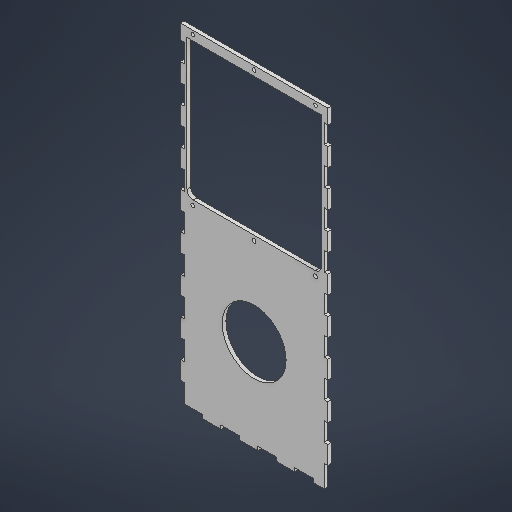
# Autodesk Inventor part: frente
Saved by Autodesk Inventor 2026 (Build 300175050, 175E)
## iProperties
Created: 2025-08-08
Part Number: frente
Material: Genérico
Document SubType Name: Modeling
Designer: EspacoMaker
Density: 1 g/cm^3
Appearance: Padrão
Author: EspacoMaker
Autodesk Inventor part; units mm, degrees
ref_plane "YZ Plane" through (0, 0, 0) normal (1, 0, 0) x (0, 1, 0)
ref_plane "XZ Plane" through (0, 0, 0) normal (0, 1, 0) x (-1, 0, 0)
ref_plane "XY Plane" through (0, 0, 0) normal (0, 0, 1) x (1, 0, 0)
sketch "Esboço1" plane through (0, 0, 0) normal (0, 0, 1) x (1, 0, 0)
  line L0 (60, -135) -> (-60, -135)
  line L1 (-60, -135) -> (-60, 135)
  line L2 (-60, 135) -> (60, 135)
  line L3 (60, 135) -> (60, -135)
  line L4 (60, -135) -> (-60, 135) construction
  line L5 (-60, -135) -> (60, 135) construction
  point P0 (0, 0)
  dimension "d0" = 120
  dimension "d1" = 270
  constraints: 12 end point, 2 midpoint, 2 parallel, 1 horizontal, 1 perpendicular
  measures "d0" distance of L1.end L2.end
  measures "d1" distance of L0.end L1.end
extrude "Extrusão1" add sketch "Esboço1" along normal blind 3
sketch "Esboço3" plane through (60, -135, 0) normal (1, 0, 0) x (0, 0, -1)
  line L0 (0, 0) -> (-3, 0) projected
  line L1 (0, 0) -> (-3, 0)
  line L2 (-3, 0) -> (-3, 18.1)
  line L3 (-3, 18.1) -> (0, 18.1)
  line L4 (0, 18.1) -> (0, 0)
  line L5 (-3, 2.9) -> (0, 2.9)
  line L6 (-3, 48.1) -> (0, 48.1)
  line L7 (-3, 32.9) -> (0, 32.9)
  line L8 (-3, 78.1) -> (0, 78.1)
  line L9 (-3, 62.9) -> (0, 62.9)
  line L10 (-3, 108.1) -> (0, 108.1)
  line L11 (-3, 92.9) -> (0, 92.9)
  line L12 (-3, 138.1) -> (0, 138.1)
  line L13 (-3, 122.9) -> (0, 122.9)
  line L14 (-3, 168.1) -> (0, 168.1)
  line L15 (-3, 152.9) -> (0, 152.9)
  line L16 (-3, 198.1) -> (0, 198.1)
  line L17 (-3, 182.9) -> (0, 182.9)
  line L18 (-3, 228.1) -> (0, 228.1)
  line L19 (-3, 212.9) -> (0, 212.9)
  line L20 (-3, 258.1) -> (0, 258.1)
  line L21 (-3, 242.9) -> (0, 242.9)
  line L22 (-3, 288.1) -> (0, 288.1)
  line L23 (-3, 272.9) -> (0, 272.9)
  line L24 (-3, 0) -> (-3, 270) projected
  line L25 (0, 0) -> (0, 270) projected
  point P0 (0, 135)
  dimension "d13" = 18.1
  dimension "d14" = 3
  dimension "d38" = 2.9
  dimension "d41" = 30
  constraints: 46 end point, 2 parallel, 2 perpendicular, 2 point on line, 1 horizontal, 1 vertical, 56 other
  measures "d13" distance of L1.end L2.end
  measures "d14" distance of L2.end L3.end
  measures "d38" distance between parallel lines of L0 L5
  measures "d41" distance of L2.end L6.start
extrude "Extrusão2" cut sketch "Esboço3" against normal blind 3 contours L0 L2 L5 L4 | L5 L2 L3 L4 | L7 L24 L6 L25 | L9 L24 L8 L25 | L11 L24 L10 L25 | L13 L24 L12 L25 | L15 L24 L14 L25 | L17 L24 L16 L25 | L19 L24 L18 L25 | L21 L24 L20 L25
sketch "Esboço5" plane through (57, -135, 0) normal (0, -1, 0) x (1, 0, 0)
  line L0 (-117, 0) -> (0, 0) projected
  line L1 (-114, 3) -> (-98.8, 3)
  line L2 (-98.8, 3) -> (-98.8, 0)
  line L3 (-98.8, 0) -> (-114, 0)
  line L4 (-114, 0) -> (-114, 3)
  line L5 (-84, 3) -> (-68.8, 3)
  line L6 (-68.8, 3) -> (-68.8, 0)
  line L7 (-68.8, 0) -> (-84, 0)
  line L8 (-84, 0) -> (-84, 3)
  line L9 (-54, 3) -> (-38.8, 3)
  line L10 (-38.8, 3) -> (-38.8, 0)
  line L11 (-38.8, 0) -> (-54, 0)
  line L12 (-54, 0) -> (-54, 3)
  line L13 (-24, 3) -> (-8.8, 3)
  line L14 (-8.8, 3) -> (-8.8, 0)
  line L15 (-8.8, 0) -> (-24, 0)
  line L16 (-24, 0) -> (-24, 3)
  line L17 (-117, 0) -> (-117, 3) projected
  point P0 (-57, 0)
  point P1 (-24, 0)
  point P2 (-54, 0)
  point P3 (-84, 0)
  point P4 (-117, 1.5)
  point P5 (-114, 1.5)
  dimension "d26" = 15.2
  dimension "d29" = 30
  dimension "d56" = 3
  constraints: 32 end point, 2 horizontal, 2 midpoint, 2 parallel, 1 collinear, 1 horizontal alignment, 1 perpendicular, 1 point on line, 23 other
  measures "d26" distance of L2.end L3.end
  measures "d29" distance of L2.end L6.end
  measures "d56" distance of point (-117, 1.5) point (-114, 1.5)
extrude "Extrusão4" cut sketch "Esboço5" against normal blind 3
sketch "Esboço7" plane through (-60, -135, 0) normal (-1, 0, 0) x (0, 0, 1)
  line L0 (3, 18.1) -> (0, 18.1) projected
  line L1 (3, 0) -> (3, 18.1) projected
  line L2 (0, 18.1) -> (0, 0) projected
  line L3 (0, 32.9) -> (3, 32.9) projected
  line L4 (3, 270) -> (3, 0) projected
  line L5 (0, 270) -> (0, 0) projected
  line L6 (0, 32.9) -> (3, 32.9)
  line L7 (0, 18.1) -> (3, 18.1)
  line L8 (0, 48.1) -> (3, 48.1)
  line L9 (0, 62.9) -> (3, 62.9)
  line L10 (0, 78.1) -> (3, 78.1)
  line L11 (0, 92.9) -> (3, 92.9)
  line L12 (0, 108.1) -> (3, 108.1)
  line L13 (0, 122.9) -> (3, 122.9)
  line L14 (0, 138.1) -> (3, 138.1)
  line L15 (0, 152.9) -> (3, 152.9)
  line L16 (0, 168.1) -> (3, 168.1)
  line L17 (0, 182.9) -> (3, 182.9)
  line L18 (0, 198.1) -> (3, 198.1)
  line L19 (0, 212.9) -> (3, 212.9)
  line L20 (0, 228.1) -> (3, 228.1)
  line L21 (0, 242.9) -> (3, 242.9)
  line L22 (0, 258.1) -> (3, 258.1)
  line L23 (0, 272.9) -> (3, 272.9)
  line L24 (0, 288.1) -> (3, 288.1)
  line L25 (0, 302.9) -> (3, 302.9)
  line L26 (3, 0) -> (0, 0) projected
  line L27 (0, 0) -> (0, 270) projected
  line L28 (0, 270) -> (3, 270) projected
  line L29 (3, 270) -> (3, 0) projected
  point P0 (0, 135)
  point P1 (3, 258.1)
  point P2 (0, 258.1)
  point P3 (0, 242.9)
  point P4 (3, 242.9)
  point P5 (3, 228.1)
  point P6 (0, 228.1)
  point P7 (0, 212.9)
  point P8 (3, 212.9)
  point P9 (3, 198.1)
  point P10 (0, 198.1)
  point P11 (0, 182.9)
  point P12 (3, 182.9)
  point P13 (3, 168.1)
  point P14 (0, 168.1)
  point P15 (0, 152.9)
  point P16 (3, 152.9)
  point P17 (3, 138.1)
  point P18 (0, 138.1)
  point P19 (0, 122.9)
  point P20 (3, 122.9)
  point P21 (3, 108.1)
  point P22 (0, 108.1)
  point P23 (0, 92.9)
  point P24 (3, 92.9)
  point P25 (3, 78.1)
  point P26 (0, 78.1)
  point P27 (0, 62.9)
  point P28 (3, 62.9)
  point P29 (3, 48.1)
  point P30 (0, 48.1)
  dimension "d49" = 30
  constraints: 40 end point, 2 horizontal, 1 vertical, 57 other
  measures "d49" distance of L0.end L8.start
extrude "Extrusão5" cut sketch "Esboço7" against normal blind 3 contours L1 L26 L2 L0 | L3 L5 L8 L4 | L9 L5 L10 L4 | L11 L5 L12 L4 | L13 L5 L14 L4 | L15 L5 L16 L4 | L17 L5 L18 L4 | L19 L5 L20 L4 | L21 L5 L22 L4
sketch "Esboço8" plane through (0, 0, 0) normal (0, 0, -1) x (-1, 0, 0)
  line L0 (-57, -86.9) -> (-60, -86.9) construction
  line L1 (-60, -86.9) -> (-60, -72.1) construction
  line L2 (-60, -72.1) -> (-57, -72.1) construction
  line L3 (-57, -72.1) -> (-57, -56.9) construction
  line L4 (-57, -56.9) -> (-60, -56.9) construction
  line L5 (-60, -56.9) -> (-60, -42.1) construction
  line L6 (-60, -42.1) -> (-57, -42.1) construction
  line L7 (-57, -42.1) -> (-57, -26.9) construction
  line L8 (-57, -26.9) -> (-60, -26.9) construction
  line L9 (-60, -26.9) -> (-60, -12.1) construction
  line L10 (-60, -12.1) -> (-57, -12.1) construction
  line L11 (-57, -12.1) -> (-57, 3.1) construction
  line L12 (-57, 3.1) -> (-60, 3.1) construction
  line L13 (-60, 3.1) -> (-60, 17.9) construction
  line L14 (-60, 17.9) -> (-57, 17.9) construction
  line L15 (-57, 17.9) -> (-57, 33.1) construction
  line L16 (-57, 33.1) -> (-60, 33.1) construction
  line L17 (-60, 33.1) -> (-60, 47.9) construction
  line L18 (-60, 47.9) -> (-57, 47.9) construction
  line L19 (-57, 47.9) -> (-57, 63.1) construction
  line L20 (-57, 63.1) -> (-60, 63.1) construction
  line L21 (-60, 63.1) -> (-60, 77.9) construction
  line L22 (-60, 77.9) -> (-57, 77.9) construction
  line L23 (-57, 77.9) -> (-57, 93.1) construction
  line L24 (-57, 93.1) -> (-60, 93.1) construction
  line L25 (-60, 93.1) -> (-60, 107.9) construction
  line L26 (-60, 107.9) -> (-57, 107.9) construction
  line L27 (-57, 107.9) -> (-57, 123.1) construction
  line L28 (-57, 123.1) -> (-60, 123.1) construction
  line L29 (-60, 123.1) -> (-60, 135) construction
  line L30 (-60, 135) -> (60, 135) construction
  line L31 (60, 135) -> (60, 123.1) construction
  line L32 (60, 123.1) -> (57, 123.1) construction
  line L33 (57, 123.1) -> (57, 107.9) construction
  line L34 (57, 107.9) -> (60, 107.9) construction
  line L35 (60, 107.9) -> (60, 93.1) construction
  line L36 (60, 93.1) -> (57, 93.1) construction
  line L37 (57, 93.1) -> (57, 77.9) construction
  line L38 (57, 77.9) -> (60, 77.9) construction
  line L39 (60, 77.9) -> (60, 63.1) construction
  line L40 (60, 63.1) -> (57, 63.1) construction
  line L41 (57, 63.1) -> (57, 47.9) construction
  line L42 (57, 47.9) -> (60, 47.9) construction
  line L43 (60, 47.9) -> (60, 33.1) construction
  line L44 (60, 33.1) -> (57, 33.1) construction
  line L45 (57, 33.1) -> (57, 17.9) construction
  line L46 (57, 17.9) -> (60, 17.9) construction
  line L47 (60, 17.9) -> (60, 3.1) construction
  line L48 (60, 3.1) -> (57, 3.1) construction
  line L49 (57, 3.1) -> (57, -12.1) construction
  line L50 (57, -12.1) -> (60, -12.1) construction
  line L51 (60, -12.1) -> (60, -26.9) construction
  line L52 (60, -26.9) -> (57, -26.9) construction
  line L53 (57, -26.9) -> (57, -42.1) construction
  line L54 (57, -42.1) -> (60, -42.1) construction
  line L55 (60, -42.1) -> (60, -56.9) construction
  line L56 (60, -56.9) -> (57, -56.9) construction
  line L57 (57, -56.9) -> (57, -72.1) construction
  line L58 (57, -72.1) -> (60, -72.1) construction
  line L59 (60, -72.1) -> (60, -86.9) construction
  line L60 (60, -86.9) -> (57, -86.9) construction
  line L61 (57, -86.9) -> (57, -102.1) construction
  line L62 (57, -102.1) -> (60, -102.1) construction
  line L63 (60, -102.1) -> (60, -116.9) construction
  line L64 (60, -116.9) -> (57, -116.9) construction
  line L65 (57, -116.9) -> (57, -132) construction
  line L66 (57, -132) -> (41.8, -132) construction
  line L67 (41.8, -132) -> (41.8, -135) construction
  line L68 (41.8, -135) -> (27, -135) construction
  line L69 (27, -135) -> (27, -132) construction
  line L70 (27, -132) -> (11.8, -132) construction
  line L71 (11.8, -132) -> (11.8, -135) construction
  line L72 (11.8, -135) -> (-3, -135) construction
  line L73 (-3, -135) -> (-3, -132) construction
  line L74 (-3, -132) -> (-18.2, -132) construction
  line L75 (-18.2, -132) -> (-18.2, -135) construction
  line L76 (-18.2, -135) -> (-33, -135) construction
  line L77 (-33, -135) -> (-33, -132) construction
  line L78 (-33, -132) -> (-48.2, -132) construction
  line L79 (-48.2, -132) -> (-48.2, -135) construction
  line L80 (-48.2, -135) -> (-57, -135) construction
  line L81 (-57, -135) -> (-57, -116.9) construction
  line L82 (-57, -116.9) -> (-60, -116.9) construction
  line L83 (-60, -116.9) -> (-60, -102.1) construction
  line L84 (-60, -102.1) -> (-57, -102.1) construction
  line L85 (-57, -102.1) -> (-57, -86.9) construction
  ellipse E0 centre (-55.4, 11.3042) end of major axis (-55.4, 8.4758) minor radius 2 (-57.4, 11.3042) -> (-57.1743, 9.9988) ccw
  line L86 (-57.1743, 9.9988) -> (59.4, 9.9988)
  line L87 (59.4, 127.5) -> (59.4, 9.9988)
  line L88 (-57.4, 127.5) -> (59.4, 127.5)
  line L89 (-57.4, 127.5) -> (-57.4, 11.3042)
  ellipse E1 centre (-56.5, 121.6939) end of major axis (-56.5, 127.5415) minor radius 2 (-54.5, 121.6939) -> (-55.7002, 127.0537) ccw
  line L90 (-55.7002, 127.0537) -> (55.7002, 127.0537)
  ellipse E2 centre (56.5, 121.6939) end of major axis (56.5, 127.5415) minor radius 2 (55.7002, 127.0537) -> (54.5, 121.6939) ccw
  line L91 (54.5, 121.6939) -> (54.5, 105.9054)
  line L92 (54.5, 105.9054) -> (49.5, 105.9054) construction
  line L93 (49.5, 105.9054) -> (49.5, 116.4119) construction
  line L94 (49.5, 116.4119) -> (-49.5, 116.4119) construction
  line L95 (-49.5, 116.4119) -> (-49.5, 105.9054) construction
  line L96 (-49.5, 105.9054) -> (-54.5, 105.9054) construction
  line L97 (-54.5, 105.9054) -> (-54.5, 121.6939)
  circle A0 centre (-50, 132) radius 1.5
  circle A1 centre (0, 132) radius 1.5
  circle A2 centre (50, 132) radius 1.5
  line L98 (60, 7.3988) -> (-60, 7.3988)
  line L99 (-60, 7.3988) -> (-60, 136)
  line L100 (-60, 136) -> (60, 136)
  line L101 (60, 136) -> (60, 7.3988)
  line L102 (-60, 7.3988) -> (60, 7.3988)
  line L103 (60, 7.3988) -> (60, 15.3988)
  line L104 (60, 15.3988) -> (-60, 15.3988)
  line L105 (-60, 15.3988) -> (-60, 7.3988)
  line L106 (-60, 11.3988) -> (60, 11.3988) construction
  circle A3 centre (0, 11.3988) radius 1.6
  circle A4 centre (-50, 11.3988) radius 1.6
  circle A5 centre (50, 11.3988) radius 1.6
  line L107 (54.5, 66.3189) -> (54.5, 124.5798)
  line L108 (-54.5, 124.5798) -> (-54.5, 66.3189)
  line L109 (-60, 136) -> (60, 136)
  line L110 (-60, 135) -> (60, 135) projected
  line L111 (-54.7, 15.3988) -> (-54.7, 127.5)
  line L112 (54.7, 127.5) -> (54.7, 15.3988)
  point P0 (-60, 49.3988)
  point P1 (54.7, 127.0537)
  point P2 (-54.7, 127.0537)
  point P3 (54.7, 124.2429)
  point P4 (-54.7, 124.2429)
  point P5 (-55.6594, 127)
  point P6 (55.6594, 127)
  point P7 (-49.2254, 9.9988)
  point P8 (-50.7746, 9.9988)
  point P9 (0.7746, 9.9988)
  point P10 (-0.7746, 9.9988)
  point P11 (50.7746, 9.9988)
  point P12 (49.2254, 9.9988)
  dimension "d91" = 8
  dimension "d92" = 3.2
  dimension "d93" = 3.2
  dimension "d94" = 3.2
  dimension "d95" = 1
  dimension "d96" = 0.2
  dimension "d97" = 0.2
  dimension "d101" = 7.5
  constraints: 52 end point, 7 point on line, 6 centre point, 5 vertical alignment, 3 midpoint, 3 parallel, 3 perpendicular, 3 vertical, 1 horizontal, 12 other
  measures "d91" distance of L102.end L104.start
  measures "d92" diameter of A4
  measures "d93" diameter of A3
  measures "d94" diameter of A5
  measures "d95" distance between parallel lines of L30 L109
  measures "d96" distance between parallel lines of L111 L108
  measures "d97" distance between parallel lines of L107 L112
  measures "d101" distance between parallel lines of L88 L30
extrude "Extrusão6" cut sketch "Esboço8" against normal up to surface (3 mm away) contours A4 L86 | L86 A4 | L111 L90 L112 L104 | L88 L112 L90 L111 | A3 L86 | L86 A3 | A5 L86 | L86 A5 | A0 | A1 | A2
fillet "Arredondamento1" radius 5 2 edges at (54.7, 15.3988, 1.5) (-54.7, 15.3988, 1.5)
sketch "Esboço9" plane through (0, 0, 0) normal (0, 0, -1) x (-1, 0, 0)
  circle A0 centre (0, -59.8006) radius 26
  line L0 (49.7, 15.3988) -> (-49.7, 15.3988) projected
  line L1 (0, 15.3988) -> (0, -135) construction
  line L2 (11.8, -135) -> (-3, -135) projected
  point P0 (0, 0)
  point P1 (0, -59.8006)
  dimension "d102" = 52
  constraints: 2 end point, 2 midpoint, 1 centre point, 1 coincident, 1 point on line, 1 vertical, 1 vertical alignment
  measures "d102" diameter of A0
extrude "Extrusão7" cut sketch "Esboço9" against normal up to surface (3 mm away)
equation "\"d14\" = d4"
equation "\"d93\" = d92"
equation "\"d94\" = d92"
equation "\"d4\" = 3"
